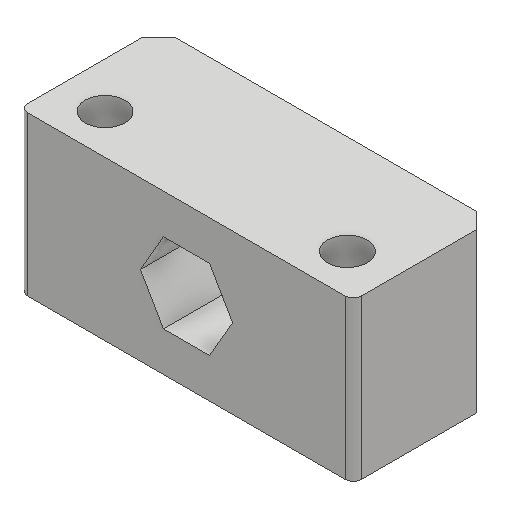
# Autodesk Inventor part: 3DP_ABS_Z_Axis_Screw_Nut_Mount
Saved by Autodesk Inventor 2026.1 (Build 301233000, 233)
## iProperties
Created: 2017-05-28
Part Number: 3DP_ABS_Z_Axis_Screw_Nut_Mount
Material: Ogólny
Document SubType Name: Modeling
Designer: Andrzej
Density: 1 g/cm^3
Appearance: Domyślna
Mass: 12.6985 g
Surface Area: 47.5511 cm^2
Volume: 12.6985 cm^3
Author: Andrzej
Autodesk Inventor part; units mm, degrees
ref_plane "YZ Plane" through (0, 0, 0) normal (1, 0, 0) x (0, 1, 0)
ref_plane "XZ Plane" through (0, 0, 0) normal (0, 1, 0) x (-1, 0, 0)
ref_plane "XY Plane" through (0, 0, 0) normal (0, 0, 1) x (1, 0, 0)
sketch "Szkic1" plane through (0, 0, 0) normal (0, 0, 1) x (1, 0, 0)
  line L0 (-6.9514, -9.6622) -> (35.0486, -9.6622)
  line L1 (35.0486, -9.6622) -> (35.0486, 7.8378)
  line L2 (35.0486, 7.8378) -> (-6.9514, 7.8378)
  line L3 (-6.9514, 7.8378) -> (-6.9514, -9.6622)
  point P0 (0, 0)
  point P1 (-1.2014, -4.6622)
  point P2 (29.2986, -4.6622)
  dimension "d0" = 42
  dimension "d1" = 17.5
  dimension "d2" = 5.75
  dimension "d3" = 5
  dimension "d4" = 5
  dimension "d5" = 5.75
  constraints: 8 end point, 2 parallel, 1 horizontal, 1 perpendicular
  measures "d0" distance of L2.end L1.end
  measures "d1" distance of L1.end L0.end
  measures "d2" distance from line of L3 point (-1.201, -4.662)
  measures "d3" distance from line of L0 point (-1.201, -4.662)
  measures "d4" distance from line of L0 point (29.299, -4.662)
  measures "d5" distance from line of L1 point (29.299, -4.662)
extrude "Wyciągnięcie proste1" add sketch "Szkic1" along normal blind 20
hole "Otwór1" at (-1.2014, -4.6622, 0) at (29.2986, -4.6622, 0) direction (0, 0, 1) diameter 5 end through all
sketch "Szkic2" plane through (-6.9514, -9.6622, 0) normal (0, -1, 0) x (1, 0, 0)
  line L0 (0, 0) -> (42, 0) projected
  line L1 (42, 0) -> (42, 20) projected
  line L2 (0, 20) -> (42, 20) projected
  line L3 (0, 0) -> (0, 20) projected
  circle A0 centre (21, 10) radius 5.025
  line L4 (23.9012, 15.025) -> (26.8024, 10)
  line L5 (26.8024, 10) -> (23.9012, 4.975)
  line L6 (23.9012, 4.975) -> (18.0988, 4.975)
  line L7 (18.0988, 4.975) -> (15.1976, 10)
  line L8 (15.1976, 10) -> (18.0988, 15.025)
  line L9 (18.0988, 15.025) -> (23.9012, 15.025)
  circle A1 centre (21, 10) radius 3.25
  point P0 (6.9514, 0)
  point P1 (21, 15.025)
  dimension "d19" = 10.05
  dimension "d15" = 42
  dimension "d16" = 20
  dimension "d17" = 10
  dimension "d18" = 21
  dimension "d20" = 6.5
  constraints: 12 end point, 3 coincident, 1 centre point, 1 midpoint, 1 vertical alignment, 15 other
  measures "d15" distance of L2.start L1.end
  measures "d16" distance of L0.start L2.start
  measures "d17" distance from line of L2 point (21, 10)
  measures "d18" distance from line of L3 point (21, 10)
  measures "d20" diameter of A1
extrude "Wyciągnięcie proste2" cut sketch "Szkic2" against normal through all contours A1
extrude "Wyciągnięcie proste3" cut sketch "Szkic2" against normal blind 10 contours A0 | A0 L4 L5 | A0 L9 L4 | L5 L6 A0 | A0 L8 L9 | L6 L7 A0 | A0 L7 L8
chamfer "Faza1" distance 0.6 angle 45 1 edges at (10.7986, 7.8378, 10)
fillet "Zaokrąglenie1" radius 1 2 edges at (-6.9514, -9.6622, 10) (35.0486, -9.6622, 10)
chamfer "Faza2" distance 2 angle 45 2 edges at (-6.9514, 7.8378, 10) (35.0486, 7.8378, 10)
equation "\"d4\" = d3"
equation "\"d5\" = d2"
equation "\"d17\" = 0.5 * d16"
equation "\"d18\" = 0.5 * d15"
